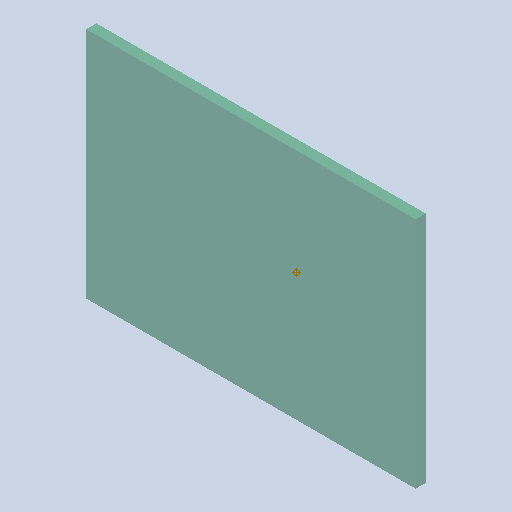
# Autodesk Inventor part: Semrock Di02-R561 dichroic beamsplitter
Saved by Autodesk Inventor 2022 (Build 260153000, 153)
## iProperties
Created: 2007-12-04
Part Number: Semrock Di02-R561 dichroic beamsplitter
Document SubType Name: Modeling
Designer: Eric Betzig
Density: 1 g/cm^3
Material: Generic
Appearance: Green (Clear)
Control State: 0
Master: False
Checked Out: False
Shininess: 20.0
Angle Display Precision: 2
Document Length Units: 11269
Document Angle Units: 11279
Document Time Units: 11290
Document Mass Units: 11283
Document Length Units Precision: 3
Document Angle Units Precision: 2
Compacted: False
Density: 0.0
Volumn: 0.0
Area: 0.0
PropertySet Name: Model Information
Author: Eric Betzig
Autodesk Inventor part; units mm, degrees
ref_plane "YZ Plane" through (0, 0, 0) normal (1, 0, 0) x (0, 1, 0)
ref_plane "XZ Plane" through (0, 0, 0) normal (0, 1, 0) x (-1, 0, 0)
sketch "Sketch1" plane through (0, 0, 0) normal (0, 0, 1) x (1, 0, 0)
  line L0 (-17.8, 12.6) -> (17.8, 12.6)
  line L1 (17.8, 12.6) -> (17.8, -12.6)
  line L2 (17.8, -12.6) -> (-17.8, -12.6)
  line L3 (-17.8, -12.6) -> (-17.8, 12.6)
  circle A0 centre (0, 0) radius 1
  dimension "d0" = 35.6
  dimension "d1" = 25.2
  dimension "d2" = 17.8
  dimension "d3" = 12.6
  constraints: 8 end point, 2 parallel, 1 centre point, 1 horizontal, 1 perpendicular, 1 other
  measures "d0" distance of L0.start L0.end
  measures "d1" distance of L2.end L0.start
  measures "d2" distance from line of A0.centre L3
  measures "d3" distance from line of A0.centre L0
extrude "Extrusion1" add sketch "Sketch1" along normal blind 1.1 contours L0 L1 L2 L3 | A0
ref_plane "Work Plane1" through (3.8, -12.6, 0) normal (1, 0, 0) x (0, 0, -1)
body "Solid1"
